Motor Coupling 8mm v5 (Autodesk Fusion 360 design; units mm, degrees)
Autodesk Fusion 360 part; units mm, degrees
sketch "Sketch1" plane through (0, 0, 0) normal (0, 0, 1) x (1, 0, 0)
  circle A0 centre (0, 0) radius 16
  circle A1 centre (0, 0) radius 12 construction
  line L0 (0, 0) -> (0, 16) construction
  circle A2 centre (0, 12) radius 2
  circle A3 centre (-12, 0) radius 2
  circle A4 centre (0, -12) radius 2
  circle A5 centre (12, 0) radius 2
  circle A6 centre (0, 0) radius 4
  dimension "d1" = 32
  dimension "d2" = 24
  dimension "d3" = 4
  dimension "d5" = 360
  dimension "d6" = 8
  constraint coincident A0.centre A1.centre
  constraint concentric A0 A1
  constraint coincident A0 L0.end
  constraint vertical L0
  constraint coincident L0 A2.centre
  measures "d1" diameter of A0
  measures "d2" diameter of A1
  measures "d3" diameter of A2
  measures "d6" diameter of A6
extrude "Extrude1" add sketch "Sketch1" along normal blind 3
sketch "Sketch2" plane through (0, 0, 3) normal (0, 0, 1) x (-1, 0, 0)
  circle A0 centre (0, -12) radius 2
  circle A1 centre (12, 0) radius 2
  circle A2 centre (0, 12) radius 2
  circle A3 centre (-12, 0) radius 2
  circle A4 centre (0, 0) radius 4
  circle A5 centre (0, 0) radius 16
  circle A6 centre (0, 0) radius 8
  dimension "d9" = 16
  constraint concentric A4 A6
  measures "d9" diameter of A6
extrude "Extrude2" add sketch "Sketch2" along normal blind 10 contours A6
ref_plane "WorkPlane1" through (5.6569, -5.6569, 11.1327) normal (0.707107, -0.707107, 0) x (-0.707107, -0.707107, 0)
sketch "Sketch3" plane through (5.6569, -5.6569, 0) normal (0.707107, -0.707107, 0) x (-0.707107, -0.707107, 0)
  line L0 (-8, -13) -> (8, -13)
  line L1 (8, -3) -> (-8, -3)
  line L2 (0, -13) -> (0, -3) construction
  circle A0 centre (0, -8) radius 2
  line L3 (0, -8) -> (0, -10)
  dimension "d13" = 4
  dimension "d14" = 3
  constraint midpoint L0 L2.start
  constraint midpoint L1 L2.end
  constraint coincident L2 A0.centre
  constraint coincident A0.centre L3.start
  constraint coincident A0 L3.end
  constraint coincident L2 L3.end
  measures "d13" diameter of A0
  measures "d14" distance of L0 L3.end
extrude "Extrude3" cut sketch "Sketch3" against normal blind 18
